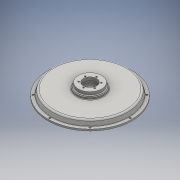
# Autodesk Inventor part: Flasque 1
Saved by Autodesk Inventor 2016 (Build 200138000, 138)
## iProperties
Created: 2015-11-14
Part Number: Flasque 1
Material: Générique
Document SubType Name: Modeling
Designer: Cyril
Density: 1 g/cm^3
Appearance: Par défaut
Author: Cyril
Autodesk Inventor part; units mm, degrees
ref_plane "YZ Plane" through (0, 0, 0) normal (1, 0, 0) x (0, 1, 0)
ref_plane "XZ Plane" through (0, 0, 0) normal (0, 1, 0) x (-1, 0, 0)
ref_plane "XY Plane" through (0, 0, 0) normal (0, 0, 1) x (1, 0, 0)
sketch "Esquisse1" plane through (0, 0, 0) normal (1, 0, 0) x (0, 1, 0)
  line L0 (0, 0) -> (0, 50.75) construction
  line L1 (102.5, -2.5) -> (106.5, -2.5)
  line L2 (106.5, -2.5) -> (106.5, 0)
  line L3 (106.5, 0) -> (115, 0)
  line L4 (115, 0) -> (115, 4.6)
  line L5 (115, 4.6) -> (106.7673, 4.6)
  line L6 (28, 34.45) -> (32, 34.45)
  line L7 (32, 34.45) -> (32, 27.15)
  line L8 (105.8014, 5.3412) -> (103.2015, 15.0441)
  arc A0 (103.2015, 15.0441) -> (98.3719, 18.75) centre (98.3719, 13.75) ccw
  line L9 (98.3719, 18.75) -> (38, 18.75)
  arc A1 (36.5, 20.25) -> (38, 18.75) centre (38, 20.25) ccw
  line L10 (36.5, 20.25) -> (36.5, 23.65)
  arc A2 (36.5, 23.65) -> (35, 25.15) centre (35, 23.65) ccw
  line L11 (35, 25.15) -> (34, 25.15)
  arc A3 (32, 27.15) -> (34, 25.15) centre (34, 27.15) ccw
  line L12 (102.5, -2.5) -> (102.5, 5.8078)
  line L13 (102.4319, 6.3254) -> (100.7057, 12.7676)
  arc A4 (105.8014, 5.3412) -> (106.7673, 4.6) centre (106.7673, 5.6) ccw
  arc A5 (102.5, 5.8078) -> (102.4319, 6.3254) centre (100.5, 5.8078) ccw
  line L14 (98.7738, 14.25) -> (40, 14.25)
  arc A6 (100.7057, 12.7676) -> (98.7738, 14.25) centre (98.7738, 12.25) ccw
  line L15 (35, 9.25) -> (35, 4.75)
  arc A7 (40, 14.25) -> (35, 9.25) centre (40, 9.25) ccw
  line L16 (34.5, 4.25) -> (32, 4.25)
  arc A8 (34.5, 4.25) -> (35, 4.75) centre (34.5, 4.75) ccw
  line L17 (32, 4.25) -> (32, 22.25)
  line L18 (32, 22.25) -> (28, 22.25)
  line L19 (28, 22.25) -> (28, 34.45)
  point P0 (106, 4.6)
  point P1 (102.5, 6.0711)
  dimension "d0" = 115
  dimension "d1" = 106.5
  dimension "d3" = 2.5
  dimension "d4" = 4.6
  dimension "d5" = 0.5
  dimension "d8" = 5
  dimension "d9" = 1.5
  dimension "d10" = 1.5
  dimension "d11" = 15.7
  dimension "d13" = 32
  dimension "d14" = 36.5
  dimension "d15" = 2
  dimension "d16" = 105
  dimension "d17" = 50.75
  dimension "d41" = 16.3
  dimension "d42" = 9.3
  dimension "d43" = 102.5
  dimension "d44" = 1
  dimension "d45" = 2
  dimension "d46" = 2
  dimension "d47" = 3
  dimension "d48" = 4.5
  dimension "d49" = 5
  dimension "d50" = 0.5
  dimension "d51" = 10
  dimension "d52" = 32
  dimension "d53" = 3
  dimension "d54" = 18
  dimension "d55" = 4
  constraints: 40 end point, 18 point on circle, 18 tangent, 9 centre point, 8 horizontal, 8 vertical, 5 point on line, 2 perpendicular, 1 parallel
  measures "d0" distance between parallel lines of L0 L4
  measures "d1" distance between parallel lines of L0 L2
  measures "d3" distance of L1.end L2.end
  measures "d4" distance of L3.end L4.end
  measures "d5" distance from line of L2 point (106, 4.6)
  measures "d8" radius of A0
  measures "d9" radius of A1
  measures "d10" radius of A2
  measures "d11" distance between parallel lines of L6 L9
  measures "d13" distance from line of L0 L6.end
  measures "d14" distance between parallel lines of L0 L10
  measures "d15" radius of A3
  measures "d16" angle of L5 L8
  measures "d17" distance of L0.start L0.end
  measures "d41" distance from line of L0.end L6
  measures "d42" distance between parallel lines of L6 L11
  measures "d43" distance between parallel lines of L0 L12
  measures "d44" radius of A4
  measures "d45" radius of A5
  measures "d46" radius of A6
  measures "d47" distance between parallel lines of L13 L8
  measures "d48" distance between parallel lines of L14 L9
  measures "d49" radius of A7
  measures "d50" radius of A8
  measures "d51" distance between parallel lines of L16 L14
  measures "d52" distance between parallel lines of L0 L17
  measures "d53" distance between parallel lines of L17 L15
  measures "d54" distance of L16.end L17.end
  measures "d55" distance of L17.end L18.end
revolve "Révolution1" add sketch "Esquisse1" angle 360 about axis through (0, 0, 0) along (0, 0, 1)
sketch "Esquisse2" plane through (0, 0, 4.6) normal (0, 0, 1) x (1, 0, 0)
  circle A0 centre (-110, 0) radius 2.65
  circle A1 centre (-77.7817, 77.7817) radius 2.65
  circle A2 centre (0, 110) radius 2.65
  circle A3 centre (77.7817, 77.7817) radius 2.65
  circle A4 centre (110, 0) radius 2.65
  circle A5 centre (77.7817, -77.7817) radius 2.65
  circle A6 centre (0, -110) radius 2.65
  circle A7 centre (-77.7817, -77.7817) radius 2.65
  line L0 (0, 0) -> (-110, 0) construction
  dimension "d19" = 5.3
  dimension "d22" = 360
  dimension "d24" = 220
  constraints: 8 centre point, 2 coincident, 2 end point, 1 horizontal, 22 other
  measures "d19" diameter of A0
  measures "d24" distance of A4.centre L0.end
extrude "Extrusion1" cut sketch "Esquisse2" against normal through all
sketch "Esquisse4" plane through (0, 0, 0) normal (1, 0, 0) x (0, 1, 0)
  line L0 (0, 0) -> (0, 50.75) construction
  line L1 (18, 34.45) -> (18, 25.45)
  line L2 (18, 25.45) -> (19.5, 25.45)
  line L3 (19.5, 25.45) -> (19.5, 18.95)
  line L4 (19.5, 18.95) -> (22, 18.95)
  line L5 (22, 18.95) -> (22, 17.15)
  line L6 (22, 17.15) -> (29, 17.15)
  line L7 (29, 17.15) -> (29, 4.45)
  line L8 (29, 4.45) -> (32, 4.45)
  line L9 (32, 4.45) -> (32, 22.45)
  line L10 (32, 22.45) -> (28, 22.45)
  line L11 (28, 22.45) -> (28, 34.45)
  line L12 (28, 34.45) -> (18, 34.45)
  dimension "d56" = 50.75
  dimension "d57" = 16.3
  dimension "d58" = 18
  dimension "d59" = 9
  dimension "d60" = 19.5
  dimension "d61" = 6.5
  dimension "d62" = 22
  dimension "d63" = 1.8
  dimension "d64" = 29
  dimension "d65" = 32
  dimension "d66" = 18
  dimension "d67" = 12
  dimension "d68" = 28
  constraints: 26 end point, 10 perpendicular, 2 vertical, 1 horizontal
  measures "d56" distance of L0.start L0.end
  measures "d57" distance from line of L12 L0.end
  measures "d58" distance between parallel lines of L0 L1
  measures "d59" distance of L1.start L1.end
  measures "d60" distance between parallel lines of L0 L3
  measures "d61" distance of L2.end L3.end
  measures "d62" distance between parallel lines of L0 L5
  measures "d63" distance of L4.end L5.end
  measures "d64" distance between parallel lines of L0 L7
  measures "d65" distance between parallel lines of L0 L9
  measures "d66" distance of L8.end L9.end
  measures "d67" distance of L10.end L11.end
  measures "d68" distance between parallel lines of L0 L11
revolve "Révolution2" add sketch "Esquisse4" angle 360 about axis through (0, 0, 0) along (0, 0, 1)
sketch "Esquisse3" plane through (0, 0, 34.45) normal (0, 0, 1) x (1, 0, 0)
  line L0 (0, 0) -> (-3.8203, 21.6658) construction
  line L1 (0, 0) -> (0, 17) construction
  circle A0 centre (0, 0) radius 17 projected
  point P0 (-20.6732, 7.5244)
  point P1 (-16.853, -14.1413)
  point P2 (3.8203, -21.6658)
  point P3 (20.6732, -7.5244)
  point P4 (16.853, 14.1413)
  dimension "d27" = 22
  dimension "d28" = 10
  dimension "d31" = 360
  constraints: 4 end point, 1 vertical, 1 vertical alignment, 8 other
  measures "d27" distance of L0.start L0.end
  measures "d28" angle of L0 L1
hole "Perçage1" at (-3.8203, 21.6658, 34.45) at (-20.6732, 7.5244, 34.45) at (-16.853, -14.1413, 34.45) at (3.8203, -21.6658, 34.45) at (20.6732, -7.5244, 34.45) at (16.853, 14.1413, 34.45) direction (0, 0, -1) diameter 4.134 end through all thread size "M5x0.8" class "6H" standard "ISO Metric profile"
